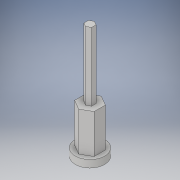
# Autodesk Inventor part: 0.5in hex to 5mm hex
Saved by Autodesk Inventor 2019 (Build 230136000, 136)
## iProperties
Created: 2020-01-30
Part Number: 0.5in hex to 5mm hex
Material: Generic
Document SubType Name: Modeling
Designer: User
Density: 1 g/cm^3
Appearance: Default
Author: User
Autodesk Inventor part; units mm, degrees
ref_plane "YZ Plane" through (0, 0, 0) normal (1, 0, 0) x (0, 1, 0)
ref_plane "XZ Plane" through (0, 0, 0) normal (0, 1, 0) x (-1, 0, 0)
ref_plane "XY Plane" through (0, 0, 0) normal (0, 0, 1) x (1, 0, 0)
sketch "Sketch1" plane through (0, 0, 0) normal (0, 1, 0) x (-1, 0, 0)
  circle A0 centre (0, 0) radius 9.525
  dimension "d0" = 19.05
  constraints: 1 centre point, 1 coincident
  measures "d0" diameter of A0
extrude "Extrusion1" add sketch "Sketch1" along normal blind 4.7625
sketch "Sketch2" plane through (0, 4.7625, 0) normal (0, 1, 0) x (1, 0, 0)
  line L0 (0, -7.3323) -> (-6.35, -3.6662)
  line L1 (-6.35, -3.6662) -> (-6.35, 3.6662)
  line L2 (-6.35, 3.6662) -> (0, 7.3323)
  line L3 (0, 7.3323) -> (6.35, 3.6662)
  line L4 (6.35, 3.6662) -> (6.35, -3.6662)
  line L5 (6.35, -3.6662) -> (0, -7.3323)
  line L6 (0, 0) -> (0, -9.525)
  circle A0 centre (0, 0) radius 9.525 projected
  dimension "d3" = 12.7
  constraints: 14 end point, 1 coincident, 1 parallel, 1 vertical, 1 vertical alignment, 14 other
  measures "d3" distance between parallel lines of L3 L0
extrude "Extrusion2" add sketch "Sketch2" along normal blind 25.4 contours L0 L1 L2 L3 L4 L5
sketch "Sketch3" plane through (0, 30.1625, 0) normal (0, 1, 0) x (1, 0, 0)
  line L0 (0, 2.8868) -> (2.5, 1.4434)
  line L1 (2.5, 1.4434) -> (2.5, -1.4434)
  line L2 (2.5, -1.4434) -> (0, -2.8868)
  line L3 (0, -2.8868) -> (-2.5, -1.4434)
  line L4 (-2.5, -1.4434) -> (-2.5, 1.4434)
  line L5 (-2.5, 1.4434) -> (0, 2.8868)
  line L6 (-6.35, -3.6662) -> (0, -7.3323) projected
  line L7 (0, 0) -> (0, -7.3323)
  dimension "d6" = 5
  constraints: 14 end point, 1 coincident, 1 parallel, 1 vertical, 13 other
  measures "d6" distance between parallel lines of L0 L3
extrude "Extrusion3" add sketch "Sketch3" along normal blind 44.45
body "Solid1"
